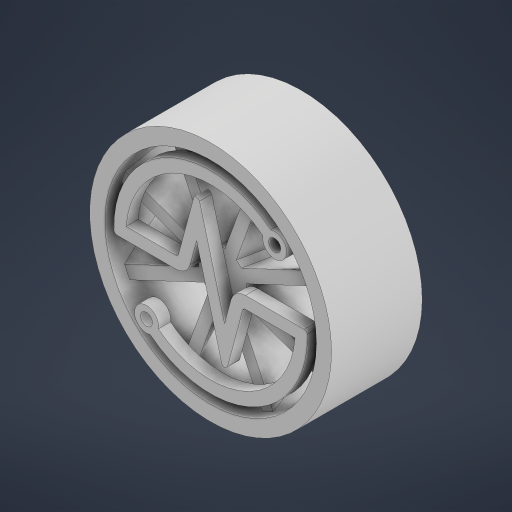
# Autodesk Inventor part: koloPredni1
Saved by Autodesk Inventor 2023 (Build 270158000, 158)
## iProperties
Created: 2024-04-14
Part Number: koloPredni1
Material: Generic
Document SubType Name: Modeling
Designer: Matooš
Density: 1 g/cm^3
Appearance: Default
Author: Matooš
Autodesk Inventor part; units mm, degrees
ref_plane "YZ Plane" through (0, 0, 0) normal (1, 0, 0) x (0, 1, 0)
ref_plane "XZ Plane" through (0, 0, 0) normal (0, 1, 0) x (-1, 0, 0)
ref_plane "XY Plane" through (0, 0, 0) normal (0, 0, 1) x (1, 0, 0)
sketch "Sketch1" plane through (0, 0, 0) normal (0, 0, 1) x (1, 0, 0)
  line L0 (0, 5.6) -> (0, -5.6) projected
  line L1 (-5.6, 0) -> (5.6, 0) projected
  circle A0 centre (0, 0) radius 4
  dimension "d0" = 8
  constraints: 2 midpoint, 1 centre point
  measures "d0" diameter of A0
extrude "Extrusion1" add sketch "Sketch1" along normal blind 13
sketch "Sketch2" plane through (0, 0, 0) normal (0, 0, 1) x (1, 0, 0)
  line L0 (0, 28) -> (0, -28) projected
  line L1 (-28, 0) -> (28, 0) projected
  circle A0 centre (0, 0) radius 20
  circle A1 centre (0, 0) radius 17.5
  dimension "d5" = 40
  dimension "d6" = 35
  constraints: 2 centre point, 2 coincident
  measures "d5" diameter of A0
  measures "d6" diameter of A1
extrude "Extrusion2" add sketch "Sketch2" along normal blind 15 contours A0 L1 A1 L0 | L0 A1 L1 A0 | A0 L0 A1 L1 | L1 A1 L0 A0
sketch "Sketch3" plane through (0, 0, 0) normal (0, 0, 1) x (1, 0, 0)
  line L0 (0, 24.5) -> (0, -24.5) projected
  line L1 (-24.5, 0) -> (24.5, 0) projected
  circle A0 centre (0, 0) radius 17.5 projected
  circle A1 centre (0, 0) radius 4 projected
  circle A2 centre (0, 0) radius 4 projected
  line L2 (-2.0315, 3.4457) -> (-11.647, 13.0613)
  circle A3 centre (0, 0) radius 17.5 projected
  line L3 (-3.4457, 2.0315) -> (-13.0613, 11.647)
  line L4 (0, 0) -> (-12.3744, 12.3744) construction
  arc A4 (-2.0315, 3.4457) -> (-3.4457, 2.0315) centre (0, 0) ccw
  arc A5 (-11.647, 13.0613) -> (-13.0613, 11.647) centre (0, 0) ccw
  dimension "d9" = 2
  dimension "d11" = 45
  constraints: 6 end point, 6 point on circle, 2 centre point, 2 coincident, 1 parallel, 8 other
  measures "d9" distance between parallel lines of L2 L3
  measures "d11" angle of L1 L4
sketch3d "3D Sketch1"
  helix H0 starts at (-7.6014, 7.6014, 0) axis through (0, 0, 0) along (0, 0, 1) pitch 185.7143 turns 0.07 hand right
sweep "Sweep1" add profiles "Sketch3" path "3D Sketch1" contours L2 A1 L3 A0
pattern_circular "Circular Pattern1" count 8 over 360 about axis through (0, 0, -10) along (0, 0, 1) of "Sweep1"
sketch "Sketch4" plane through (0, 0, 13) normal (0, 0, 1) x (1, 0, 0)
  line L0 (-13.9642, 1) -> (-5.3955, 1)
  line L1 (-5.3955, 1) -> (-2.3141, 12.5)
  line L2 (-2.3141, 12.5) -> (2.3141, -4.7726)
  line L3 (2.3141, -4.7726) -> (3.8609, 1)
  line L4 (3.8609, 1) -> (15.9687, 1)
  line L5 (-15.9687, -1) -> (-3.8609, -1)
  line L6 (-3.8609, -1) -> (-2.3141, 4.7726)
  line L7 (-2.3141, 4.7726) -> (2.3141, -12.5)
  line L8 (2.3141, -12.5) -> (5.3955, -1)
  line L9 (5.3955, -1) -> (13.9642, -1)
  line L10 (-16, 0) -> (16, 0) construction
  line L11 (0, 16) -> (0, -16) construction
  line L12 (0, 29.3239) -> (0, -29.3239) projected
  line L13 (-28.506, 0) -> (28.506, 0) projected
  line L14 (-10.6066, -10.6066) -> (10.6066, 10.6066) construction
  line L15 (11.3137, -11.3137) -> (-11.3137, 11.3137) construction
  arc A0 (-8.6477, -11.0099) -> (-9.9801, -12.5059) centre (-10.6066, -10.6066) ccw
  circle A1 centre (-10.6066, -10.6066) radius 1
  circle A2 centre (0, 0) radius 15 construction
  arc A3 (8.6477, 11.0099) -> (9.9801, 12.5059) centre (10.6066, 10.6066) ccw
  circle A4 centre (10.6066, 10.6066) radius 1
  arc A5 (-8.6477, -11.0099) -> (13.9642, -1) centre (0, 0) ccw
  arc A6 (-9.9801, -12.5059) -> (15.9687, 1) centre (0, 0) ccw
  arc A7 (9.9801, 12.5059) -> (-15.9687, -1) centre (0, 0) ccw
  arc A8 (8.6477, 11.0099) -> (-13.9642, 1) centre (0, 0) ccw
  point P0 (-16, 0)
  point P1 (-3.5929, 0)
  point P2 (16, 0)
  point P3 (3.5929, 0)
  dimension "d22" = 2
  dimension "d23" = 2
  dimension "d24" = 2
  dimension "d26" = 105
  dimension "d27" = 2
  dimension "d28" = 75
  dimension "d29" = 1
  dimension "d30" = 45
  dimension "d31" = 4
  dimension "d32" = 2
  dimension "d34" = 30
  dimension "d35" = 4
  dimension "d36" = 2
  dimension "d37" = 2
  dimension "d38" = 1
  dimension "d39" = 1
  dimension "d40" = 25
  dimension "d41" = 12.5
  constraints: 28 end point, 20 point on circle, 10 midpoint, 9 centre point, 5 coincident, 4 parallel, 3 collinear, 2 horizontal, 2 point on line, 1 perpendicular, 2 other
  measures "d22" distance between parallel lines of L0 L5
  measures "d23" distance between parallel lines of L1 L6
  measures "d24" distance between parallel lines of L2 L7
  measures "d26" angle of L0 L1
  measures "d27" distance between parallel lines of L3 L8
  measures "d28" angle of L10 L7
  measures "d29" distance from line of L2 point (0, 0)
  measures "d30" angle of L14 L11
  measures "d31" diameter of A0
  measures "d32" diameter of A1
  measures "d34" diameter of A2
  measures "d35" diameter of A3
  measures "d36" diameter of A4
  measures "d37" radial gap between concentric circles of A6 A5
  measures "d38" radial gap between concentric circles of A5 A2
  measures "d39" radial gap between concentric circles of A2 A8
  measures "d40" vertical distance of L1.end L7.end
  measures "d41" distance from line of L10 L1.end
extrude "Extrusion3" add sketch "Sketch4" along normal blind 2 contours L0 L1 L2 L12 L13 L7 L6 A7 A8 | L12 A7 A3 A8 | L2 L13 L12 | L13 L6 L5 A7 | L2 L3 L13 A6 L12 A5 L9 L8 L7 | L12 L7 L13 | L3 L4 A6 L13 | L12 A6 A0 A5
fillet "Fillet1" radius 0.5 6 edges at (-2.3141, 12.5, 14) (2.3141, -12.5, 14) (5.3955, -1, 14) (-5.3955, 1, 14) (-15.9687, -1, 14) (15.9687, 1, 14)
fillet "Fillet2" radius 2.5 2 edges at (3.8609, 1, 14) (-3.8609, -1, 14)
sketch "Sketch6" plane through (0, 0, 0) normal (0, 0, -1) x (1, 0, 0)
  line L0 (0, 28) -> (0, -28) projected
  line L1 (28, 0) -> (-28, 0) projected
  circle A0 centre (0, 0) radius 7.05
  dimension "d60" = 14.1
  constraints: 1 centre point, 1 coincident
  measures "d60" diameter of A0
extrude "Extrusion5" cut sketch "Sketch6" against normal blind 4.5
sketch "Sketch7" plane through (0, 0, 4.5) normal (0, 0, -1) x (1, 0, 0)
  line L0 (28, 0) -> (-28, 0) projected
  line L1 (0, 28) -> (0, -28) projected
  circle A0 centre (0, 0) radius 7.05
  circle A1 centre (0, 0) radius 5.05
  dimension "d61" = 14.1
  dimension "d62" = 10.1
  constraints: 2 centre point, 2 coincident
  measures "d61" diameter of A0
  measures "d62" diameter of A1
extrude "Extrusion6" add sketch "Sketch7" along normal blind 4.5 contours A0 L1 A1 L0 | L0 A1 L1 A0 | L1 A1 L0 A0 | A0 L0 A1 L1
body "Solid1"
